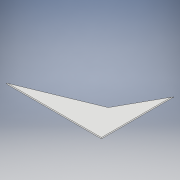
# Autodesk Inventor part: Rocket_MK_II_Fins_II
Saved by Autodesk Inventor 2017 (Build 210142000, 142)
## iProperties
Created: 2017-05-01
Part Number: Rocket_MK_II_Fins_II
Material: ABS Plastic
Document SubType Name: Modeling
Designer: Harrison
Density: 1.06 g/cm^3
Appearance: Smooth - White
Mass: 3.34374 g
Surface Area: 53.3653 cm^2
Volume: 3.15447 cm^3
Author: Harrison
Autodesk Inventor part; units mm, degrees
ref_plane "YZ Plane" through (0, 0, 0) normal (1, 0, 0) x (0, 1, 0)
ref_plane "XZ Plane" through (0, 0, 0) normal (0, 1, 0) x (-1, 0, 0)
ref_plane "XY Plane" through (0, 0, 0) normal (0, 0, 1) x (1, 0, 0)
sketch "Sketch1" plane through (0, 0, 0) normal (0, 1, 0) x (-1, 0, 0)
  line L0 (0, 0) -> (101.6, 0)
  line L1 (0, 0) -> (0, -76.2)
  line L2 (101.6, 0) -> (24.8951, -31.5247)
  line L3 (24.8951, -31.5247) -> (0, -76.2)
  dimension "d0" = 101.6
  dimension "d1" = 76.2
  constraints: 8 end point, 1 horizontal, 1 vertical
  measures "d0" distance of L0.start L0.end
  measures "d1" distance of L0.start L1.end
extrude "Extrusion1" add sketch "Sketch1" along normal blind 1.27
chamfer "Chamfer1" distance 0.635 angle 45 2 edges at (-12.4476, 1.27, -53.8624) (-63.2476, 1.27, -15.7624)
chamfer "Chamfer2" distance 0.635 angle 45 2 edges at (-12.4476, 0, -53.8624) (-63.2476, 0, -15.7624)
chamfer "Chamfer3" distance 0.635 angle 45 1 edges at (0, 1.27, -37.4477)
chamfer "Chamfer4" distance 0.635 angle 45 1 edges at (0, 0, -37.4483)
body "Solid1"
